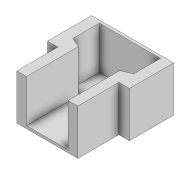
# Autodesk Inventor part: large_room1
Saved by Autodesk Inventor 2021 (Build 250183000, 183)
## iProperties
Created: 2022-05-19
Part Number: large_room1
Material: Generic
Document SubType Name: Modeling
Designer: Derm
Density: 1 g/cm^3
Appearance: Default
Author: Derm
Autodesk Inventor part; units mm, degrees
ref_plane "YZ Plane" through (0, 0, 0) normal (1, 0, 0) x (0, 1, 0)
ref_plane "XZ Plane" through (0, 0, 0) normal (0, 1, 0) x (-1, 0, 0)
ref_plane "XY Plane" through (0, 0, 0) normal (0, 0, 1) x (1, 0, 0)
sketch "Sketch1" plane through (0, 0, 0) normal (0, 1, 0) x (-1, 0, 0)
  line L0 (0, 0) -> (0, -14.0125) construction
  line L1 (12.3617, 25.4) -> (12.3617, -5.3655)
  line L2 (12.3617, -5.3655) -> (18.1749, -5.3655)
  line L3 (18.1844, -7.8927) -> (18.1844, -25.4)
  line L4 (18.1749, 25.4) -> (18.1749, 0.9638)
  line L5 (18.1749, 0.9638) -> (24.4214, 0.9638)
  line L6 (24.4214, 0.9638) -> (24.4214, -25.4)
  line L7 (18.1749, 25.4) -> (12.3617, 25.4)
  line L8 (18.1844, -25.4) -> (24.4214, -25.4)
  line L9 (-12.3617, 25.4) -> (-12.3617, -5.3655)
  line L10 (-12.3617, -5.3655) -> (-18.1749, 9.6342)
  line L11 (-18.1844, -7.8927) -> (-18.1844, -25.4)
  line L12 (-18.1749, 25.4) -> (-18.1749, 0.9638)
  line L13 (-18.1749, 0.9638) -> (-24.4214, 0.9638)
  line L14 (-24.4214, 0.9638) -> (-24.4214, -25.4)
  line L15 (-18.1749, 25.4) -> (-12.3617, 25.4)
  line L16 (-18.1844, -25.4) -> (-24.4214, -25.4)
  line L17 (12.3617, -5.3655) -> (18.1844, -7.8927)
  line L18 (-12.3617, -5.3655) -> (-18.1844, -7.8927)
  line L19 (12.3617, -5.3655) -> (0, 0) construction
  line L20 (27.1198, 0) -> (23.5153, 0) construction
  point P0 (18.1938, 0)
  point P1 (-18.1938, 0)
  point P2 (25.3175, 0)
  dimension "d10" = 50.8
  dimension "d11" = 25.4
  constraints: 42 end point, 9 symmetric about line, 4 perpendicular, 3 horizontal, 2 point on line, 2 vertical, 1 collinear, 1 midpoint, 1 other
  measures "d10" distance from line of L3.end L7
  measures "d11" distance from line of L0.start L7
extrude "Extrusion1" add sketch "Sketch1" against normal mid plane 25.4
sketch "Sketch2" plane through (0, -12.7, 0) normal (0, -1, 0) x (1, 0, 0)
  line L0 (-12.3617, -5.3655) -> (-12.3617, 25.4) projected
  line L1 (-12.3617, 25.4) -> (-18.1749, 25.4) projected
  line L2 (-18.1749, 25.4) -> (-18.1749, 0.9638) projected
  line L3 (-18.1749, 0.9638) -> (-24.4214, 0.9638) projected
  line L4 (-24.4214, 0.9638) -> (-24.4214, -25.4) projected
  line L5 (-24.4214, -25.4) -> (-18.1844, -25.4) projected
  line L6 (-18.1844, -25.4) -> (-18.1844, -7.8927) projected
  line L7 (24.4214, 0.9638) -> (18.1749, 0.9638) projected
  line L8 (18.1749, 0.9638) -> (18.1749, 25.4) projected
  line L9 (18.1749, 25.4) -> (12.3617, 25.4) projected
  line L10 (12.3617, 25.4) -> (12.3617, -5.3655) projected
  line L11 (18.1844, -7.8927) -> (18.1844, -25.4) projected
  line L12 (18.1844, -25.4) -> (24.4214, -25.4) projected
  line L13 (24.4214, -25.4) -> (24.4214, 0.9638) projected
  line L14 (18.1749, 25.4) -> (12.3617, 25.4) projected
  line L15 (-12.3617, 25.4) -> (-18.1749, 25.4) projected
  line L16 (18.1749, 25.4) -> (-18.1749, 25.4)
  line L17 (24.4214, 0.9638) -> (24.4214, -25.4) projected
  line L18 (24.4214, -25.4) -> (-24.4214, -25.4)
  line L19 (12.3617, -5.3655) -> (18.1844, -7.8927) projected
  line L20 (-18.1844, -7.8927) -> (-12.3617, -5.3655) projected
  point P0 (0, 0)
  constraints: 4 end point, 1 horizontal, 1 perpendicular
extrude "Extrusion2" add sketch "Sketch2" along normal blind 1.5875
sketch "Sketch4" plane through (0, -12.7, 0) normal (0, 1, 0) x (1, 0, 0)
  line L0 (18.1844, 7.8927) -> (18.1844, 25.4) projected
  line L1 (-18.1844, 25.4) -> (18.1844, 25.4) projected
  line L2 (-18.1844, 25.4) -> (-18.1844, 7.8927) projected
  line L3 (-18.1844, 7.8927) -> (-12.3617, 5.3655) projected
  line L4 (-12.3617, 5.3655) -> (-12.3617, -25.4) projected
  line L5 (12.3617, -25.4) -> (-12.3617, -25.4) projected
  line L6 (12.3617, -25.4) -> (12.3617, 5.3655) projected
  line L7 (12.3617, 5.3655) -> (18.1844, 7.8927) projected
  line L8 (-18.1844, 25.4) -> (18.1844, 25.4)
  line L9 (18.1844, 25.4) -> (18.1844, 23.7858)
  line L10 (18.1844, 23.7858) -> (-18.1844, 23.7858)
  line L11 (-18.1844, 23.7858) -> (-18.1844, 25.4)
  point P0 (0, 0)
  constraints: 8 end point, 2 parallel, 1 horizontal, 1 perpendicular, 1 point on line
extrude "Extrusion4" add sketch "Sketch4" along normal up to surface (25.4 mm away) contours L10 L2 L1 L0
body "Solid1"
